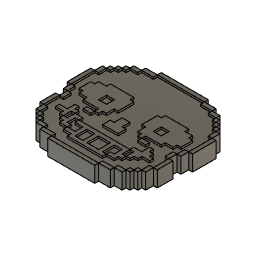
sans v1 (Autodesk Fusion 360 design; units mm, degrees)
Autodesk Fusion 360 part; units mm, degrees
note: some values were not read from the file. Chosen so that the rebuilt part matches the saved one: which bodies a step acts on.
sketch "Sketch1" plane through (0, 0, 0) normal (0, 0, 1) x (1, 0, 0)
  line L0 (0, 10) -> (6, 10)
  line L1 (6, 10) -> (6, 8)
  line L2 (6, 8) -> (10, 8)
  line L3 (10, 8) -> (10, 6)
  line L4 (10, 6) -> (12, 6)
  line L5 (12, 6) -> (12, 4)
  line L6 (12, 4) -> (14, 4)
  line L7 (14, 4) -> (14, 2)
  line L8 (14, 2) -> (16, 2)
  line L9 (16, 2) -> (16, 0)
  line L10 (16, 0) -> (18, 0)
  line L11 (18, 0) -> (18, -4)
  line L12 (18, -4) -> (20, -4)
  line L13 (20, -4) -> (20, -16)
  line L14 (20, -16) -> (18, -16)
  line L15 (18, -16) -> (18, -20)
  line L16 (18, -20) -> (16, -20)
  line L17 (16, -20) -> (16, -24)
  line L18 (16, -24) -> (18, -24)
  line L19 (18, -24) -> (18, -32)
  line L20 (18, -32) -> (16, -32)
  line L21 (16, -32) -> (16, -36)
  line L22 (16, -36) -> (14, -36)
  line L23 (14, -36) -> (14, -38)
  line L24 (14, -38) -> (12, -38)
  line L25 (12, -38) -> (12, -40)
  line L26 (12, -40) -> (10, -40)
  line L27 (10, -40) -> (10, -42)
  line L28 (10, -42) -> (6, -42)
  line L29 (6, -42) -> (6, -44)
  line L30 (6, -44) -> (0, -44)
  line L31 (0, -44) -> (0, -46)
  line L32 (0, -46) -> (-24, -46)
  line L33 (-24, -46) -> (-24, -44)
  line L34 (-24, -44) -> (-30, -44)
  line L35 (-30, -44) -> (-30, -42)
  line L36 (-30, -42) -> (-34, -42)
  line L37 (-34, -42) -> (-34, -40)
  line L38 (-34, -40) -> (-36, -40)
  line L39 (-36, -40) -> (-36, -38)
  line L40 (-36, -38) -> (-38, -38)
  line L41 (-38, -38) -> (-38, -36)
  line L42 (-38, -36) -> (-40, -36)
  line L43 (-40, -36) -> (-40, -32)
  line L44 (-40, -32) -> (-42, -32)
  line L45 (-42, -32) -> (-42, -24)
  line L46 (-42, -24) -> (-40, -24)
  line L47 (-40, -24) -> (-40, -20)
  line L48 (-40, -20) -> (-42, -20)
  line L49 (-42, -20) -> (-42, -16)
  line L50 (-42, -16) -> (-44, -16)
  line L51 (-44, -16) -> (-44, -4)
  line L52 (-44, -4) -> (-42, -4)
  line L53 (-42, -4) -> (-42, 0)
  line L54 (-42, 0) -> (-40, 0)
  line L55 (-40, 0) -> (-40, 2)
  line L56 (-40, 2) -> (-38, 2)
  line L57 (-38, 2) -> (-38, 4)
  line L58 (-38, 4) -> (-36, 4)
  line L59 (-36, 4) -> (-36, 6)
  line L60 (-36, 6) -> (-34, 6)
  line L61 (-34, 6) -> (-34, 8)
  line L62 (-34, 8) -> (-30, 8)
  line L63 (-30, 8) -> (-30, 10)
  line L64 (-30, 10) -> (-24, 10)
  line L65 (-24, 10) -> (-24, 12)
  line L66 (-24, 12) -> (0, 12)
  line L67 (0, 12) -> (0, 10)
  constraint horizontal L0
  constraint perpendicular L0 L1
  constraint perpendicular L1 L2
  constraint perpendicular L2 L3
  constraint perpendicular L3 L4
  constraint perpendicular L4 L5
  constraint perpendicular L5 L6
  constraint perpendicular L6 L7
  constraint perpendicular L7 L8
  constraint perpendicular L8 L9
  constraint perpendicular L9 L10
  constraint perpendicular L10 L11
  constraint perpendicular L11 L12
  constraint perpendicular L12 L13
  constraint perpendicular L13 L14
  constraint perpendicular L14 L15
  constraint perpendicular L15 L16
  constraint perpendicular L16 L17
  constraint perpendicular L17 L18
  constraint perpendicular L18 L19
  constraint perpendicular L19 L20
  constraint perpendicular L20 L21
  constraint perpendicular L21 L22
  constraint perpendicular L22 L23
  constraint perpendicular L23 L24
  constraint perpendicular L24 L25
  constraint perpendicular L25 L26
  constraint perpendicular L26 L27
  constraint perpendicular L27 L28
  constraint perpendicular L28 L29
  constraint perpendicular L29 L30
  constraint perpendicular L30 L31
  constraint perpendicular L31 L32
  constraint perpendicular L32 L33
  constraint perpendicular L33 L34
  constraint perpendicular L34 L35
  constraint perpendicular L35 L36
  constraint perpendicular L36 L37
  constraint perpendicular L37 L38
  constraint perpendicular L38 L39
  constraint perpendicular L39 L40
  constraint perpendicular L40 L41
  constraint perpendicular L41 L42
  constraint perpendicular L42 L43
  constraint perpendicular L43 L44
  constraint perpendicular L44 L45
  constraint perpendicular L45 L46
  constraint perpendicular L46 L47
  constraint perpendicular L47 L48
  constraint perpendicular L48 L49
  constraint perpendicular L49 L50
  constraint perpendicular L50 L51
  constraint perpendicular L51 L52
  constraint perpendicular L52 L53
  constraint perpendicular L53 L54
  constraint perpendicular L54 L55
  constraint perpendicular L55 L56
  constraint perpendicular L56 L57
  constraint perpendicular L57 L58
  constraint perpendicular L58 L59
  constraint perpendicular L59 L60
  constraint perpendicular L60 L61
  constraint perpendicular L61 L62
  constraint perpendicular L62 L63
  constraint perpendicular L63 L64
  constraint perpendicular L64 L65
  constraint perpendicular L65 L66
  constraint perpendicular L0 L67
extrude "Extrude1" add sketch "Sketch1" along normal blind 7 makes body 1
sketch "Sketch2" plane through (0, 0, 7) normal (0, 0, 1) x (-1, 0, 0)
  line L0 (0, -12) -> (24, -12)
  line L1 (24, -12) -> (24, -10)
  line L2 (24, -10) -> (30, -10)
  line L3 (30, -10) -> (30, -8)
  line L4 (30, -8) -> (34, -8)
  line L5 (34, -8) -> (34, -6)
  line L6 (34, -6) -> (36, -6)
  line L7 (36, -6) -> (36, -4)
  line L8 (36, -4) -> (38, -4)
  line L9 (38, -4) -> (38, -2)
  line L10 (38, -2) -> (40, -2)
  line L11 (40, -2) -> (40, 0)
  line L12 (40, 0) -> (42, 0)
  line L13 (42, 0) -> (42, 4)
  line L14 (42, 4) -> (44, 4)
  line L15 (44, 4) -> (44, 16)
  line L16 (44, 16) -> (42, 16)
  line L17 (42, 16) -> (42, 20)
  line L18 (42, 20) -> (40, 20)
  line L19 (40, 20) -> (40, 24)
  line L20 (40, 24) -> (42, 24)
  line L21 (42, 24) -> (42, 32)
  line L22 (42, 32) -> (40, 32)
  line L23 (40, 32) -> (40, 36)
  line L24 (40, 36) -> (38, 36)
  line L25 (38, 36) -> (38, 38)
  line L26 (38, 38) -> (36, 38)
  line L27 (36, 38) -> (36, 40)
  line L28 (36, 40) -> (34, 40)
  line L29 (34, 40) -> (34, 42)
  line L30 (34, 42) -> (30, 42)
  line L31 (30, 42) -> (30, 44)
  line L32 (30, 44) -> (24, 44)
  line L33 (24, 44) -> (24, 46)
  line L34 (24, 46) -> (0, 46)
  line L35 (0, 46) -> (0, 44)
  line L36 (0, 44) -> (-6, 44)
  line L37 (-6, 44) -> (-6, 42)
  line L38 (-6, 42) -> (-10, 42)
  line L39 (-10, 42) -> (-10, 40)
  line L40 (-10, 40) -> (-12, 40)
  line L41 (-12, 40) -> (-12, 38)
  line L42 (-12, 38) -> (-14, 38)
  line L43 (-14, 38) -> (-14, 36)
  line L44 (-14, 36) -> (-16, 36)
  line L45 (-16, 36) -> (-16, 32)
  line L46 (-16, 32) -> (-18, 32)
  line L47 (-18, 32) -> (-18, 24)
  line L48 (-18, 24) -> (-16, 24)
  line L49 (-16, 24) -> (-16, 20)
  line L50 (-16, 20) -> (-18, 20)
  line L51 (-18, 20) -> (-18, 16)
  line L52 (-18, 16) -> (-20, 16)
  line L53 (-20, 16) -> (-20, 4)
  line L54 (-20, 4) -> (-18, 4)
  line L55 (-18, 4) -> (-18, 0)
  line L56 (-18, 0) -> (-16, 0)
  line L57 (-16, 0) -> (-16, -2)
  line L58 (-16, -2) -> (-14, -2)
  line L59 (-14, -2) -> (-14, -4)
  line L60 (-14, -4) -> (-12, -4)
  line L61 (-12, -4) -> (-12, -6)
  line L62 (-12, -6) -> (-10, -6)
  line L63 (-10, -6) -> (-10, -8)
  line L64 (-10, -8) -> (-6, -8)
  line L65 (-6, -8) -> (-6, -10)
  line L66 (-6, -10) -> (0, -10)
  line L67 (0, -10) -> (0, -12)
  line L68 (24, -12) -> (0, -12)
  line L69 (0, -12) -> (0, -10)
  line L70 (0, -10) -> (24, -10)
  line L71 (24, -10) -> (24, -12)
  line L72 (0, -10) -> (-6, -10)
  line L73 (-6, -10) -> (-6, -8)
  line L74 (-6, -8) -> (0, -8)
  line L75 (0, -8) -> (0, -10)
  line L76 (-6, -8) -> (-10, -8)
  line L77 (-10, -8) -> (-10, -6)
  line L78 (-10, -6) -> (-6, -6)
  line L79 (-6, -6) -> (-6, -8)
  line L80 (-10, -6) -> (-12, -6)
  line L81 (-12, -6) -> (-12, -4)
  line L82 (-12, -4) -> (-10, -4)
  line L83 (-10, -4) -> (-10, -6)
  line L84 (-12, -4) -> (-14, -4)
  line L85 (-14, -4) -> (-14, -2)
  line L86 (-14, -2) -> (-12, -2)
  line L87 (-12, -2) -> (-12, -4)
  line L88 (-14, -2) -> (-16, -2)
  line L89 (-16, -2) -> (-16, 0)
  line L90 (-16, 0) -> (-14, 0)
  line L91 (-14, 0) -> (-14, -2)
  line L92 (-16, 0) -> (-18, 0)
  line L93 (-18, 0) -> (-18, 4)
  line L94 (-18, 4) -> (-16, 4)
  line L95 (-16, 4) -> (-16, 0)
  line L96 (-18, 4) -> (-20, 4)
  line L97 (-20, 4) -> (-20, 16)
  line L98 (-20, 16) -> (-18, 16)
  line L99 (-18, 16) -> (-18, 4)
  line L100 (-18, 16) -> (-16, 16)
  line L101 (-16, 16) -> (-16, 20)
  line L102 (-16, 20) -> (-18, 20)
  line L103 (-18, 20) -> (-18, 16)
  line L104 (-16, 20) -> (-14, 20)
  line L105 (-14, 20) -> (-14, 24)
  line L106 (-14, 24) -> (-16, 24)
  line L107 (-16, 24) -> (-16, 20)
  line L108 (-16, 24) -> (-18, 24)
  line L109 (-18, 24) -> (-18, 32)
  line L110 (-18, 32) -> (-16, 32)
  line L111 (-16, 32) -> (-16, 24)
  line L112 (-16, 32) -> (-14, 32)
  line L113 (-14, 32) -> (-14, 36)
  line L114 (-14, 36) -> (-16, 36)
  line L115 (-16, 36) -> (-16, 32)
  line L116 (-14, 36) -> (-12, 36)
  line L117 (-12, 36) -> (-12, 38)
  line L118 (-12, 38) -> (-14, 38)
  line L119 (-14, 38) -> (-14, 36)
  line L120 (-12, 38) -> (-10, 38)
  line L121 (-10, 38) -> (-10, 40)
  line L122 (-10, 40) -> (-12, 40)
  line L123 (-12, 40) -> (-12, 38)
  line L124 (-10, 40) -> (-6, 40)
  line L125 (-6, 40) -> (-6, 42)
  line L126 (-6, 42) -> (-10, 42)
  line L127 (-10, 42) -> (-10, 40)
  line L128 (-6, 42) -> (0, 42)
  line L129 (0, 42) -> (0, 44)
  line L130 (0, 44) -> (-6, 44)
  line L131 (-6, 44) -> (-6, 42)
  line L132 (0, 44) -> (24, 44)
  line L133 (24, 44) -> (24, 46)
  line L134 (24, 46) -> (0, 46)
  line L135 (0, 46) -> (0, 44)
  line L136 (24, 44) -> (30, 44)
  line L137 (30, 44) -> (30, 42)
  line L138 (30, 42) -> (24, 42)
  line L139 (24, 42) -> (24, 44)
  line L140 (30, 42) -> (34, 42)
  line L141 (34, 42) -> (34, 40)
  line L142 (34, 40) -> (30, 40)
  line L143 (30, 40) -> (30, 42)
  line L144 (34, 40) -> (36, 40)
  line L145 (36, 40) -> (36, 38)
  line L146 (36, 38) -> (34, 38)
  line L147 (34, 38) -> (34, 40)
  line L148 (36, 38) -> (38, 38)
  line L149 (38, 38) -> (38, 36)
  line L150 (38, 36) -> (36, 36)
  line L151 (36, 36) -> (36, 38)
  line L152 (38, 36) -> (40, 36)
  line L153 (40, 36) -> (40, 32)
  line L154 (40, 32) -> (38, 32)
  line L155 (38, 32) -> (38, 36)
  line L156 (40, 32) -> (42, 32)
  line L157 (42, 32) -> (42, 24)
  line L158 (42, 24) -> (40, 24)
  line L159 (40, 24) -> (40, 32)
  line L160 (40, 24) -> (38, 24)
  line L161 (38, 24) -> (38, 20)
  line L162 (38, 20) -> (40, 20)
  line L163 (40, 20) -> (40, 24)
  line L164 (40, 20) -> (42, 20)
  line L165 (42, 20) -> (42, 16)
  line L166 (42, 16) -> (40, 16)
  line L167 (40, 16) -> (40, 20)
  line L168 (42, 16) -> (44, 16)
  line L169 (44, 16) -> (44, 4)
  line L170 (44, 4) -> (42, 4)
  line L171 (42, 4) -> (42, 16)
  line L172 (42, 4) -> (40, 4)
  line L173 (40, 4) -> (40, 0)
  line L174 (40, 0) -> (42, 0)
  line L175 (42, 0) -> (42, 4)
  line L176 (40, 0) -> (38, 0)
  line L177 (38, 0) -> (38, -2)
  line L178 (38, -2) -> (40, -2)
  line L179 (40, -2) -> (40, 0)
  line L180 (36, -4) -> (38, -4)
  line L181 (38, -4) -> (38, -2)
  line L182 (38, -2) -> (36, -2)
  line L183 (36, -2) -> (36, -4)
  line L184 (36, -4) -> (34, -4)
  line L185 (34, -4) -> (34, -6)
  line L186 (34, -6) -> (36, -6)
  line L187 (36, -6) -> (36, -4)
  line L188 (34, -6) -> (30, -6)
  line L189 (30, -6) -> (30, -8)
  line L190 (30, -8) -> (34, -8)
  line L191 (34, -8) -> (34, -6)
  line L192 (30, -8) -> (24, -8)
  line L193 (24, -8) -> (24, -10)
  line L194 (24, -10) -> (30, -10)
  line L195 (30, -10) -> (30, -8)
  constraint horizontal L68
  constraint vertical L69
  constraint horizontal L70
  constraint vertical L71
  constraint coincident L66.end L67.start
  constraint coincident L0.end L1.start
  constraint horizontal L72
  constraint vertical L73
  constraint horizontal L74
  constraint vertical L75
  constraint coincident L64.end L65.start
  constraint horizontal L76
  constraint vertical L77
  constraint horizontal L78
  constraint vertical L79
  constraint coincident L62.end L63.start
  constraint horizontal L80
  constraint vertical L81
  constraint horizontal L82
  constraint vertical L83
  constraint coincident L60.end L61.start
  constraint horizontal L84
  constraint vertical L85
  constraint horizontal L86
  constraint vertical L87
  constraint coincident L58.end L59.start
  constraint horizontal L88
  constraint vertical L89
  constraint horizontal L90
  constraint vertical L91
  constraint coincident L56.end L57.start
  constraint horizontal L92
  constraint vertical L93
  constraint horizontal L94
  constraint vertical L95
  constraint coincident L54.end L55.start
  constraint horizontal L96
  constraint vertical L97
  constraint horizontal L98
  constraint vertical L99
  constraint coincident L52.end L53.start
  constraint horizontal L100
  constraint vertical L101
  constraint horizontal L102
  constraint vertical L103
  constraint coincident L49.end L50.start
  constraint horizontal L104
  constraint vertical L105
  constraint horizontal L106
  constraint vertical L107
  constraint horizontal L108
  constraint vertical L109
  constraint horizontal L110
  constraint vertical L111
  constraint coincident L46.end L47.start
  constraint coincident L48.end L49.start
  constraint horizontal L112
  constraint vertical L113
  constraint horizontal L114
  constraint vertical L115
  constraint coincident L43.end L44.start
  constraint coincident L45.end L46.start
  constraint horizontal L116
  constraint vertical L117
  constraint horizontal L118
  constraint vertical L119
  constraint coincident L41.end L42.start
  constraint horizontal L120
  constraint vertical L121
  constraint horizontal L122
  constraint vertical L123
  constraint coincident L39.end L40.start
  constraint horizontal L124
  constraint vertical L125
  constraint horizontal L126
  constraint vertical L127
  constraint coincident L37.end L38.start
  constraint horizontal L128
  constraint vertical L129
  constraint horizontal L130
  constraint vertical L131
  constraint coincident L35.end L36.start
  constraint horizontal L132
  constraint vertical L133
  constraint horizontal L134
  constraint vertical L135
  constraint coincident L33.end L34.start
  constraint horizontal L136
  constraint vertical L137
  constraint horizontal L138
  constraint vertical L139
  constraint coincident L30.end L31.start
  constraint coincident L32.end L33.start
  constraint horizontal L140
  constraint vertical L141
  constraint horizontal L142
  constraint vertical L143
  constraint coincident L28.end L29.start
  constraint horizontal L144
  constraint vertical L145
  constraint horizontal L146
  constraint vertical L147
  constraint coincident L26.end L27.start
  constraint horizontal L148
  constraint vertical L149
  constraint horizontal L150
  constraint vertical L151
  constraint coincident L24.end L25.start
  constraint horizontal L152
  constraint vertical L153
  constraint horizontal L154
  constraint vertical L155
  constraint coincident L22.end L23.start
  constraint horizontal L156
  constraint vertical L157
  constraint horizontal L158
  constraint vertical L159
  constraint coincident L20.end L21.start
  constraint horizontal L160
  constraint vertical L161
  constraint horizontal L162
  constraint vertical L163
  constraint horizontal L164
  constraint vertical L165
  constraint horizontal L166
  constraint vertical L167
  constraint coincident L16.end L17.start
  constraint horizontal L168
  constraint vertical L169
  constraint horizontal L170
  constraint vertical L171
  constraint coincident L14.end L15.start
  constraint horizontal L172
  constraint vertical L173
  constraint horizontal L174
  constraint vertical L175
  constraint coincident L11.end L12.start
  constraint horizontal L176
  constraint vertical L177
  constraint horizontal L178
  constraint vertical L179
  constraint coincident L9.end L10.start
  constraint horizontal L180
  constraint vertical L181
  constraint horizontal L182
  constraint vertical L183
  constraint coincident L7.end L8.start
  constraint horizontal L184
  constraint vertical L185
  constraint horizontal L186
  constraint vertical L187
  constraint coincident L5.end L6.start
  constraint horizontal L188
  constraint vertical L189
  constraint horizontal L190
  constraint vertical L191
  constraint coincident L3.end L4.start
  constraint horizontal L192
  constraint vertical L193
  constraint horizontal L194
  constraint vertical L195
  constraint coincident L1.end L2.start
extrude "Extrude2" add sketch "Sketch2" along normal blind 1 separate body contours L0 L1 L67 L68 L69 L70 L71 | L65 L66 L72 L73 L74 L75 | L2 L3 L192 L193 L194 L195 | L63 L64 L76 L77 L78 L79 | L4 L5 L188 L189 L190 L191 | L61 L62 L80 L81 L82 L83 | L6 L7 L184 L185 L186 L187 | L59 L60 L84 L85 L86 L87 | L8 L9 L180 L181 L182 L183 | L57 L58 L88 L89 L90 L91 | L10 L11 L176 L177 L178 L179 | L55 L56 L92 L93 L94 L95 | L12 L13 L172 L173 L174 L175 | L52 L53 L54 L96 L97 L98 L99 | L14 L15 L16 L168 L169 L170 L171 | L50 L51 L100 L101 L102 L103 | L17 L18 L164 L165 L166 L167 | L49 L104 L105 L106 L107 | L19 L160 L161 L162 L163 | L46 L47 L48 L108 L109 L110 L111 | L20 L21 L22 L156 L157 L158 L159 | L44 L45 L112 L113 L114 L115 | L23 L24 L152 L153 L154 L155 | L42 L43 L116 L117 L118 L119 | L25 L26 L148 L149 L150 L151 | L40 L41 L120 L121 L122 L123 | L27 L28 L144 L145 L146 L147 | L38 L39 L124 L125 L126 L127 | L29 L30 L140 L141 L142 L143 | L36 L37 L128 L129 L130 L131 | L31 L32 L136 L137 L138 L139 | L33 L34 L35 L132 L133 L134 L135 makes body 2 at (-26, 8.6667, 7)
sketch "Sketch3" plane through (0, 0, 7) normal (0, 0, 1) x (-1, 0, 0)
  line L0 (0, -12) -> (24, -12)
  line L1 (24, -12) -> (24, -10)
  line L2 (24, -10) -> (30, -10)
  line L3 (30, -10) -> (30, -8)
  line L4 (30, -8) -> (34, -8)
  line L5 (34, -8) -> (34, -6)
  line L6 (34, -6) -> (36, -6)
  line L7 (36, -6) -> (36, -4)
  line L8 (36, -4) -> (38, -4)
  line L9 (38, -4) -> (38, -2)
  line L10 (38, -2) -> (40, -2)
  line L11 (40, -2) -> (40, 0)
  line L12 (40, 0) -> (42, 0)
  line L13 (42, 0) -> (42, 4)
  line L14 (42, 4) -> (44, 4)
  line L15 (44, 4) -> (44, 16)
  line L16 (44, 16) -> (42, 16)
  line L17 (42, 16) -> (42, 20)
  line L18 (42, 20) -> (40, 20)
  line L19 (40, 20) -> (40, 24)
  line L20 (40, 24) -> (42, 24)
  line L21 (42, 24) -> (42, 32)
  line L22 (42, 32) -> (40, 32)
  line L23 (40, 32) -> (40, 36)
  line L24 (40, 36) -> (38, 36)
  line L25 (38, 36) -> (38, 38)
  line L26 (38, 38) -> (36, 38)
  line L27 (36, 38) -> (36, 40)
  line L28 (36, 40) -> (34, 40)
  line L29 (34, 40) -> (34, 42)
  line L30 (34, 42) -> (30, 42)
  line L31 (30, 42) -> (30, 44)
  line L32 (30, 44) -> (24, 44)
  line L33 (24, 44) -> (24, 46)
  line L34 (24, 46) -> (0, 46)
  line L35 (0, 46) -> (0, 44)
  line L36 (0, 44) -> (-6, 44)
  line L37 (-6, 44) -> (-6, 42)
  line L38 (-6, 42) -> (-10, 42)
  line L39 (-10, 42) -> (-10, 40)
  line L40 (-10, 40) -> (-12, 40)
  line L41 (-12, 40) -> (-12, 38)
  line L42 (-12, 38) -> (-14, 38)
  line L43 (-14, 38) -> (-14, 36)
  line L44 (-14, 36) -> (-16, 36)
  line L45 (-16, 36) -> (-16, 32)
  line L46 (-16, 32) -> (-18, 32)
  line L47 (-18, 32) -> (-18, 24)
  line L48 (-18, 24) -> (-16, 24)
  line L49 (-16, 24) -> (-16, 20)
  line L50 (-16, 20) -> (-18, 20)
  line L51 (-18, 20) -> (-18, 16)
  line L52 (-18, 16) -> (-20, 16)
  line L53 (-20, 16) -> (-20, 4)
  line L54 (-20, 4) -> (-18, 4)
  line L55 (-18, 4) -> (-18, 0)
  line L56 (-18, 0) -> (-16, 0)
  line L57 (-16, 0) -> (-16, -2)
  line L58 (-16, -2) -> (-14, -2)
  line L59 (-14, -2) -> (-14, -4)
  line L60 (-14, -4) -> (-12, -4)
  line L61 (-12, -4) -> (-12, -6)
  line L62 (-12, -6) -> (-10, -6)
  line L63 (-10, -6) -> (-10, -8)
  line L64 (-10, -8) -> (-6, -8)
  line L65 (-6, -8) -> (-6, -10)
  line L66 (-6, -10) -> (0, -10)
  line L67 (0, -10) -> (0, -12)
  line L68 (38, 16) -> (38, 10)
  line L69 (38, 10) -> (36, 10)
  line L70 (36, 10) -> (36, 8)
  line L71 (36, 8) -> (32, 8)
  line L72 (38, 16) -> (36, 16)
  line L73 (36, 16) -> (36, 18)
  line L74 (36, 18) -> (32, 18)
  line L75 (32, 18) -> (32, 20)
  line L76 (32, 20) -> (24, 20)
  line L77 (24, 20) -> (24, 22)
  line L78 (24, 22) -> (22, 22)
  line L79 (22, 22) -> (22, 20)
  line L80 (22, 20) -> (20, 20)
  line L81 (20, 20) -> (20, 16)
  line L82 (20, 16) -> (18, 16)
  line L83 (18, 16) -> (18, 8)
  line L84 (18, 8) -> (20, 8)
  line L85 (20, 8) -> (20, 6)
  line L86 (20, 6) -> (32, 6)
  line L87 (32, 6) -> (32, 8)
  line L88 (24, 22) -> (28, 22)
  line L89 (28, 22) -> (28, 24)
  line L90 (28, 24) -> (24, 24)
  line L91 (24, 24) -> (24, 22)
  line L92 (24, 16) -> (28, 16)
  line L93 (28, 16) -> (28, 12)
  line L94 (28, 12) -> (24, 12)
  line L95 (24, 12) -> (24, 16)
  line L96 (16, 22) -> (14, 22)
  line L97 (14, 22) -> (14, 18)
  line L98 (14, 18) -> (10, 18)
  line L99 (10, 18) -> (10, 22)
  line L100 (10, 22) -> (8, 22)
  line L101 (8, 22) -> (8, 26)
  line L102 (8, 26) -> (16, 26)
  line L103 (16, 26) -> (16, 22)
  line L104 (6, 16) -> (6, 8)
  line L105 (6, 8) -> (4, 8)
  line L106 (4, 8) -> (4, 6)
  line L107 (4, 6) -> (-8, 6)
  line L108 (-8, 6) -> (-8, 8)
  line L109 (-8, 8) -> (-12, 8)
  line L110 (-12, 8) -> (-12, 10)
  line L111 (-12, 10) -> (-14, 10)
  line L112 (-14, 10) -> (-14, 16)
  line L113 (-14, 16) -> (-12, 16)
  line L114 (-12, 16) -> (-12, 18)
  line L115 (-12, 18) -> (-8, 18)
  line L116 (-8, 18) -> (-8, 20)
  line L117 (-8, 20) -> (0, 20)
  line L118 (0, 20) -> (0, 22)
  line L119 (0, 22) -> (2, 22)
  line L120 (2, 22) -> (2, 20)
  line L121 (2, 20) -> (4, 20)
  line L122 (4, 20) -> (4, 16)
  line L123 (4, 16) -> (6, 16)
  line L124 (0, 16) -> (0, 12)
  line L125 (0, 12) -> (-4, 12)
  line L126 (-4, 12) -> (-4, 16)
  line L127 (-4, 16) -> (0, 16)
  line L128 (0, 22) -> (0, 24)
  line L129 (0, 24) -> (-4, 24)
  line L130 (-4, 24) -> (-4, 22)
  line L131 (-4, 22) -> (0, 22)
  line L132 (30, 24) -> (32, 24)
  line L133 (32, 24) -> (32, 28)
  line L134 (32, 28) -> (36, 28)
  line L135 (36, 28) -> (36, 30)
  line L136 (36, 30) -> (32, 30)
  line L137 (32, 30) -> (32, 32)
  line L138 (32, 32) -> (30, 32)
  line L139 (30, 32) -> (30, 28)
  line L140 (30, 28) -> (28, 28)
  line L141 (28, 28) -> (28, 26)
  line L142 (28, 26) -> (30, 26)
  line L143 (30, 26) -> (30, 24)
  line L144 (30, 32) -> (28, 32)
  line L145 (28, 32) -> (28, 28)
  line L146 (30, 32) -> (30, 34)
  line L147 (30, 34) -> (28, 34)
  line L148 (28, 34) -> (28, 36)
  line L149 (28, 36) -> (24, 36)
  line L150 (24, 36) -> (24, 34)
  line L151 (24, 34) -> (26, 34)
  line L152 (26, 34) -> (26, 30)
  line L153 (26, 30) -> (24, 30)
  line L154 (24, 30) -> (24, 28)
  line L155 (28, 28) -> (24, 28)
  line L156 (24, 36) -> (24, 38)
  line L157 (24, 38) -> (20, 38)
  line L158 (24, 36) -> (20, 36)
  line L159 (20, 36) -> (20, 32)
  line L160 (20, 32) -> (24, 32)
  line L161 (24, 32) -> (24, 30)
  line L162 (24, 30) -> (14, 30)
  line L163 (18, 32) -> (18, 38)
  line L164 (18, 38) -> (14, 38)
  line L165 (14, 38) -> (14, 32)
  line L166 (14, 32) -> (18, 32)
  line L167 (12, 32) -> (12, 38)
  line L168 (12, 38) -> (6, 38)
  line L169 (6, 38) -> (6, 32)
  line L170 (6, 32) -> (12, 32)
  line L171 (4, 32) -> (4, 38)
  line L172 (4, 38) -> (2, 38)
  line L173 (2, 38) -> (2, 36)
  line L174 (2, 36) -> (0, 36)
  line L175 (0, 36) -> (0, 32)
  line L176 (0, 32) -> (4, 32)
  line L177 (20, 38) -> (20, 40)
  line L178 (20, 40) -> (2, 40)
  line L179 (2, 40) -> (2, 38)
  line L180 (2, 38) -> (-2, 38)
  line L181 (-2, 38) -> (-2, 36)
  line L182 (-2, 36) -> (-4, 36)
  line L183 (-4, 36) -> (-4, 34)
  line L184 (-4, 34) -> (-2, 34)
  line L185 (-2, 34) -> (-2, 30)
  line L186 (-2, 30) -> (14, 30)
  line L187 (-2, 30) -> (-4, 30)
  line L188 (-4, 30) -> (-4, 34)
  line L189 (-2, 30) -> (-2, 28)
  line L190 (-2, 28) -> (-6, 28)
  line L191 (-6, 28) -> (-6, 24)
  line L192 (-6, 24) -> (-8, 24)
  line L193 (-8, 24) -> (-8, 26)
  line L194 (-8, 26) -> (-10, 26)
  line L195 (-10, 26) -> (-10, 28)
  line L196 (-10, 28) -> (-12, 28)
  line L197 (-12, 28) -> (-12, 30)
  line L198 (-12, 30) -> (-8, 30)
  line L199 (-8, 30) -> (-8, 32)
  line L200 (-8, 32) -> (-6, 32)
  line L201 (-6, 32) -> (-6, 34)
  line L202 (-6, 34) -> (-4, 34)
  constraint vertical L68
  constraint perpendicular L68 L69
  constraint perpendicular L69 L70
  constraint perpendicular L70 L71
  constraint perpendicular L68 L72
  constraint perpendicular L72 L73
  constraint perpendicular L73 L74
  constraint perpendicular L74 L75
  constraint perpendicular L75 L76
  constraint perpendicular L76 L77
  constraint perpendicular L77 L78
  constraint perpendicular L78 L79
  constraint perpendicular L79 L80
  constraint perpendicular L80 L81
  constraint perpendicular L81 L82
  constraint perpendicular L82 L83
  constraint perpendicular L83 L84
  constraint perpendicular L84 L85
  constraint perpendicular L85 L86
  constraint perpendicular L71 L87
  constraint perpendicular L77 L88
  constraint perpendicular L88 L89
  constraint perpendicular L89 L90
  constraint perpendicular L78 L91
  constraint perpendicular L79 L92
  constraint perpendicular L92 L93
  constraint perpendicular L93 L94
  constraint perpendicular L92 L95
  constraint perpendicular L83 L96
  constraint perpendicular L96 L97
  constraint perpendicular L97 L98
  constraint perpendicular L98 L99
  constraint perpendicular L99 L100
  constraint perpendicular L100 L101
  constraint perpendicular L101 L102
  constraint perpendicular L96 L103
  constraint perpendicular L96 L104
  constraint perpendicular L104 L105
  constraint perpendicular L105 L106
  constraint perpendicular L106 L107
  constraint perpendicular L107 L108
  constraint perpendicular L108 L109
  constraint perpendicular L109 L110
  constraint perpendicular L110 L111
  constraint perpendicular L111 L112
  constraint perpendicular L112 L113
  constraint perpendicular L113 L114
  constraint perpendicular L114 L115
  constraint perpendicular L115 L116
  constraint perpendicular L116 L117
  constraint perpendicular L117 L118
  constraint perpendicular L118 L119
  constraint perpendicular L119 L120
  constraint perpendicular L120 L121
  constraint perpendicular L121 L122
  constraint perpendicular L104 L123
  constraint perpendicular L117 L124
  constraint perpendicular L124 L125
  constraint perpendicular L125 L126
  constraint perpendicular L124 L127
  constraint perpendicular L119 L128
  constraint perpendicular L128 L129
  constraint perpendicular L129 L130
  constraint perpendicular L128 L131
  constraint perpendicular L97 L132
  constraint perpendicular L132 L133
  constraint perpendicular L133 L134
  constraint perpendicular L134 L135
  constraint perpendicular L135 L136
  constraint perpendicular L136 L137
  constraint perpendicular L137 L138
  constraint perpendicular L138 L139
  constraint perpendicular L139 L140
  constraint perpendicular L140 L141
  constraint perpendicular L141 L142
  constraint perpendicular L132 L143
  constraint perpendicular L139 L144
  constraint perpendicular L140 L145
  constraint perpendicular L144 L146
  constraint perpendicular L146 L147
  constraint perpendicular L147 L148
  constraint perpendicular L148 L149
  constraint perpendicular L149 L150
  constraint perpendicular L150 L151
  constraint perpendicular L151 L152
  constraint perpendicular L152 L153
  constraint perpendicular L153 L154
  constraint perpendicular L154 L155
  constraint perpendicular L149 L156
  constraint perpendicular L156 L157
  constraint perpendicular L156 L158
  constraint perpendicular L158 L159
  constraint perpendicular L159 L160
  constraint perpendicular L153 L161
  constraint perpendicular L161 L162
  constraint perpendicular L162 L163
  constraint perpendicular L163 L164
  constraint perpendicular L164 L165
  constraint perpendicular L163 L166
  constraint perpendicular L164 L167
  constraint perpendicular L167 L168
  constraint perpendicular L168 L169
  constraint perpendicular L167 L170
  constraint perpendicular L170 L171
  constraint perpendicular L171 L172
  constraint perpendicular L172 L173
  constraint perpendicular L173 L174
  constraint perpendicular L174 L175
  constraint perpendicular L171 L176
  constraint perpendicular L157 L177
  constraint perpendicular L177 L178
  constraint perpendicular L172 L179
  constraint perpendicular L179 L180
  constraint perpendicular L180 L181
  constraint perpendicular L181 L182
  constraint perpendicular L182 L183
  constraint perpendicular L183 L184
  constraint perpendicular L184 L185
  constraint perpendicular L185 L186
  constraint perpendicular L185 L187
  constraint perpendicular L184 L188
  constraint perpendicular L186 L189
  constraint perpendicular L189 L190
  constraint perpendicular L190 L191
  constraint perpendicular L191 L192
  constraint perpendicular L192 L193
  constraint perpendicular L193 L194
  constraint perpendicular L194 L195
  constraint perpendicular L195 L196
  constraint perpendicular L196 L197
  constraint perpendicular L197 L198
  constraint perpendicular L198 L199
  constraint perpendicular L199 L200
  constraint perpendicular L200 L201
  constraint perpendicular L183 L202
extrude "Extrude3" add sketch "Sketch3" along normal blind 1 separate body contours L88 L89 L90 L91 | L68 L69 L70 L71 L72 L73 L74 L75 L76 L77 L78 L79 L80 L81 L82 L83 L84 L85 L86 L87 | L96 L97 L98 L99 L100 L101 L102 L103 | L128 L129 L130 L131 | L104 L105 L106 L107 L108 L109 L110 L111 L112 L113 L114 L115 L116 L117 L118 L119 L120 L121 L122 L123 | L132 L133 L134 L135 L136 L137 L138 L139 L140 L141 L142 L143 | L144 L145 L146 L147 L148 L149 L150 L151 L152 L153 L154 L155 | L156 L157 L158 L159 L160 L161 L162 L177 L178 L179 L180 L181 L182 L183 L184 L185 L186 | L187 L188 L189 L190 L191 L192 L193 L194 L195 L196 L197 L198 L199 L200 L201 L202 makes body 3 at (-26.6667, -8, 7) makes body 3 at (-25.3333, -23.3333, 7) makes body 4 at (-31.3333, -26, 7) makes body 4 at (-26, -28.6667, 7) makes body 4 at (-11.3333, -30.6667, 7) makes body 4 at (6.6667, -26, 7) makes body 5 at (1.3333, -8, 7) makes body 5 at (1.3333, -22.6667, 7) makes body 6 at (-12.6667, -24.6667, 7)
combine "Combine1" operation add target body 1 tool bodies 2
combine "Combine2" operation add target body 1 tool bodies 3 5 6 4
